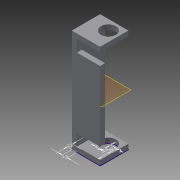
# Autodesk Inventor part: Lifter
Saved by Autodesk Inventor 2014 SP1 (Build 180222100, 222)
## iProperties
Created: 2015-03-30
Part Number: Lifter
Material: Generic
Document SubType Name: Modeling
Designer: Erin
Density: 1 g/cm^3
Appearance: Default
Author: Erin
Autodesk Inventor part; units mm, degrees
ref_plane "YZ Plane" through (0, 0, 0) normal (1, 0, 0) x (0, 1, 0)
ref_plane "XZ Plane" through (0, 0, 0) normal (0, 1, 0) x (-1, 0, 0)
sketch "Sketch1" plane through (0, 0, 0) normal (0, 0, 1) x (1, 0, 0)
  circle A0 centre (0, 0) radius 2.25
  line L0 (-4, 3) -> (3, 3)
  line L1 (3, 3) -> (3, -4)
  line L2 (3, -4) -> (-4, -4)
  line L3 (-4, -4) -> (-4, 3)
  line L4 (-4, 3) -> (-5.5, 3)
  line L5 (-5.5, 3) -> (-5.5, -5.5)
  line L6 (-5.5, -5.5) -> (-4, -5.5)
  line L7 (-4, -5.5) -> (-4, 3)
  line L8 (3, -4) -> (-4, -4)
  line L9 (-4, -4) -> (-4, -5.5)
  line L10 (-4, -5.5) -> (3, -5.5)
  line L11 (3, -5.5) -> (3, -4)
  dimension "d0" = 4.5
  dimension "d1" = 4
  dimension "d2" = 4
  dimension "d3" = 3
  dimension "d5" = 3
  dimension "d6" = 1.5
  dimension "d7" = 1.5
  constraints: 24 end point, 6 parallel, 3 horizontal, 3 perpendicular, 2 collinear, 1 centre point, 1 coincident
  measures "d0" diameter of A0
  measures "d1" distance from line of A0.centre L2
  measures "d2" distance from line of A0.centre L3
  measures "d3" distance from line of A0.centre L0
  measures "d5" distance from line of A0.centre L1
  measures "d6" distance of L6.end L5.end
  measures "d7" distance of L9.end L8.end
extrude "Extrusion1" add sketch "Sketch1" along normal blind 1.5
extrude "Extrusion2" add sketch "Sketch1" along normal blind 29.5 contours L3 L7 L6 L5 L4 | L2 L11 L10 L7
ref_plane "Work Plane2" through (0, 0, 15.5) normal (0, 0, 1) x (1, 0, 0)
mirror "Mirror2" about plane through (0, 0, 15.5) normal (0, 0, 1) of "Extrusion1"
sketch "Sketch2" plane through (-4, -4, 1.5) normal (0, 1, 0) x (1, 0, 0)
  line L0 (7, 0) -> (7, -28) projected
  line L1 (0, 0) -> (7, 0)
  line L2 (7, 0) -> (7, -3.5)
  line L3 (7, -3.5) -> (0, -3.5)
  line L4 (0, -3.5) -> (0, 0)
  point P0 (4, 1.5)
  dimension "d13" = 3.5
  constraints: 8 end point, 2 parallel, 1 horizontal, 1 perpendicular, 1 point on line
  measures "d13" distance of L1.end L2.end
extrude "Extrusion3" cut sketch "Sketch2" against normal blind 10
mirror "Mirror3" about plane through (0, 0, 15.5) normal (0, 0, 1) of "Extrusion3"
body "Solid1"
